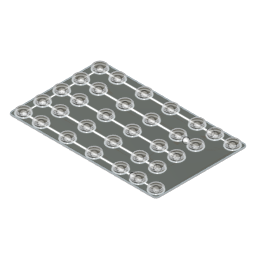
heliumv0.0.1prototype (Autodesk Fusion 360 design; units mm, degrees)
Autodesk Fusion 360 part; units mm, degrees
note: some values were not read from the file. Set by a fixed rule: which sketch regions a step uses.
sketch "Sketch1" plane through (0, 0, 0) normal (0, 0, 1) x (1, 0, 0)
  line L0 (2, 0) -> (98, 0)
  line L1 (100, 2) -> (100, 60)
  line L2 (98, 62) -> (2, 62)
  line L3 (0, 60) -> (0, 2)
  arc A0 (2, 62) -> (0, 60) centre (2, 60) ccw
  arc A1 (100, 60) -> (98, 62) centre (98, 60) ccw
  arc A2 (98, 0) -> (100, 2) centre (98, 2) ccw
  arc A3 (0, 2) -> (2, 0) centre (2, 2) ccw
  point P0 (100, 0)
  point P1 (0, 62)
  dimension "d1" = 100
  dimension "d2" = 62
  dimension "d3" = 2
  constraint horizontal L0
  constraint vertical L1
  constraint horizontal L2
  constraint vertical L3
  constraint coincident P1 L2
  constraint coincident P1 L3
  constraint tangent L2 A0
  constraint tangent L3 A0
  constraint tangent L1 A1
  constraint tangent L2 A1
  constraint equal A0 A1
  constraint coincident P0 L0
  constraint coincident P0 L1
  constraint tangent L0 A2
  constraint tangent L1 A2
  constraint equal A0 A2
  constraint coincident origin L0
  constraint coincident origin L3
  constraint tangent L0 A3
  constraint tangent L3 A3
  constraint equal A0 A3
  measures "d1" distance of origin P0
  measures "d2" distance of origin P1
  measures "d3" radius of A0
extrude "Extrude1" add sketch "Sketch1" along normal blind 0.5
sketch "Sketch2" plane through (0, 0, 0.5) normal (0, 0, 1) x (-1, 0, 0)
  arc A0 (0, -2) -> (-2, 0) centre (-2, -2) ccw
  line L0 (-2, 0) -> (-98, 0)
  arc A1 (-98, 0) -> (-100, -2) centre (-98, -2) ccw
  line L1 (-100, -2) -> (-100, -60)
  arc A2 (-100, -60) -> (-98, -62) centre (-98, -60) ccw
  line L2 (-98, -62) -> (-2, -62)
  arc A3 (-2, -62) -> (0, -60) centre (-2, -60) ccw
  line L3 (0, -60) -> (0, -2)
  line L4 (-5, -44) -> (-76.5418, -44)
  line L5 (-5, -44) -> (-17, -44)
  circle A4 centre (-5, -44) radius 4
  circle A5 centre (-17, -44) radius 4
  line L6 (-17, -44) -> (-35, -44)
  circle A6 centre (-35, -44) radius 4
  line L7 (-35, -44) -> (-40.411, -44)
  line L8 (-35, -44) -> (-53, -44)
  circle A7 centre (-53, -44) radius 4
  line L9 (-53, -44) -> (-59.411, -44)
  line L10 (-53, -44) -> (-71, -44)
  circle A8 centre (-71, -44) radius 4
  line L11 (-71, -44) -> (-83, -44)
  circle A9 centre (-83, -44) radius 4
  line L12 (-5, -44) -> (-5, -57)
  line L13 (-5, -57) -> (-79.7487, -57)
  circle A10 centre (-5, -57) radius 4
  line L14 (-5, -57) -> (-17, -57)
  line L15 (-17, -57) -> (-35, -57)
  line L16 (-35, -57) -> (-53, -57)
  line L17 (-53, -57) -> (-71, -57)
  line L18 (-71, -57) -> (-83, -57)
  circle A11 centre (-17, -57) radius 4
  circle A12 centre (-35, -57) radius 4
  circle A13 centre (-53, -57) radius 4
  circle A14 centre (-71, -57) radius 4
  circle A15 centre (-83, -57) radius 4
  line L19 (-5, -44) -> (-5, -31)
  line L20 (-5, -31) -> (-5, -18)
  circle A16 centre (-5, -31) radius 4
  circle A17 centre (-5, -18) radius 4
  line L21 (-5, -18) -> (-5, -5)
  circle A18 centre (-5, -5) radius 4
  line L22 (-5, -31) -> (-6.411, -31)
  line L23 (-6.411, -31) -> (-80.411, -31)
  line L24 (-5, -18) -> (-79.9028, -18)
  line L25 (-5, -5) -> (-79.411, -5)
  line L26 (-5, -31) -> (-17, -31)
  line L27 (-5, -18) -> (-17, -18)
  line L28 (-17, -31) -> (-17.411, -31)
  line L29 (-17, -31) -> (-35, -31)
  line L30 (-35, -31) -> (-53, -31)
  line L31 (-53, -31) -> (-71, -31)
  line L32 (-71, -31) -> (-83, -31)
  line L33 (-17, -18) -> (-35, -18)
  line L34 (-35, -18) -> (-53, -18)
  line L35 (-53, -18) -> (-71, -18)
  line L36 (-71, -18) -> (-83, -18)
  line L37 (-5, -5) -> (-17, -5)
  line L38 (-17, -5) -> (-35, -5)
  line L39 (-35, -5) -> (-53, -5)
  line L40 (-53, -5) -> (-71, -5)
  line L41 (-71, -5) -> (-83, -5)
  circle A19 centre (-17, -31) radius 4
  circle A20 centre (-35, -31) radius 4
  circle A21 centre (-53, -31) radius 4
  circle A22 centre (-71, -31) radius 4
  circle A23 centre (-83, -31) radius 4
  circle A24 centre (-83, -18) radius 4
  circle A25 centre (-71, -18) radius 4
  circle A26 centre (-53, -18) radius 4
  circle A27 centre (-35, -18) radius 4
  circle A28 centre (-17, -18) radius 4
  circle A29 centre (-17, -5) radius 4
  circle A30 centre (-35, -5) radius 4
  circle A31 centre (-53, -5) radius 4
  circle A32 centre (-71, -5) radius 4
  circle A33 centre (-83, -5) radius 4
  line L42 (-83, -5) -> (-95, -5)
  circle A34 centre (-95, -5) radius 4
  line L43 (-79.7487, -57) -> (-80, -57)
  line L44 (-83, -57) -> (-95, -57)
  circle A35 centre (-95, -57) radius 4
  dimension "d6" = 12
  dimension "d7" = 8
  dimension "d8" = 8
  dimension "d9" = 18
  dimension "d10" = 8
  dimension "d11" = 18
  dimension "d12" = 8
  dimension "d13" = 18
  dimension "d14" = 8
  dimension "d15" = 12
  dimension "d16" = 8
  dimension "d17" = 13
  dimension "d18" = 8
  dimension "d19" = 12
  dimension "d20" = 18
  dimension "d21" = 18
  dimension "d22" = 18
  dimension "d23" = 12
  dimension "d24" = 8
  dimension "d25" = 8
  dimension "d26" = 8
  dimension "d27" = 8
  dimension "d28" = 8
  dimension "d29" = 13
  dimension "d30" = 13
  dimension "d31" = 8
  dimension "d32" = 8
  dimension "d33" = 13
  dimension "d34" = 8
  dimension "d35" = 12
  dimension "d36" = 12
  dimension "d37" = 18
  dimension "d38" = 18
  dimension "d39" = 18
  dimension "d40" = 12
  dimension "d41" = 18
  dimension "d42" = 18
  dimension "d43" = 18
  dimension "d44" = 12
  dimension "d45" = 12
  dimension "d46" = 18
  dimension "d47" = 18
  dimension "d48" = 18
  dimension "d49" = 12
  dimension "d50" = 8
  dimension "d51" = 8
  dimension "d52" = 8
  dimension "d53" = 8
  dimension "d54" = 8
  dimension "d55" = 8
  dimension "d56" = 8
  dimension "d57" = 8
  dimension "d58" = 8
  dimension "d59" = 8
  dimension "d60" = 8
  dimension "d61" = 8
  dimension "d62" = 8
  dimension "d63" = 8
  dimension "d64" = 8
  dimension "d65" = 12
  dimension "d66" = 8
  dimension "d67" = 5
  dimension "d68" = 5
  dimension "d76" = 12
  dimension "d77" = 8
  constraint horizontal L4
  constraint perpendicular L3 L5
  constraint coincident L4.start L5.start
  constraint coincident L5.end A5.centre
  constraint parallel L4 L6
  constraint coincident L6.end A6.centre
  constraint coincident L4 L7.end
  constraint parallel L4 L7
  constraint parallel L4 L8
  constraint coincident L8.end A7.centre
  constraint coincident L4 L9.end
  constraint parallel L4 L10
  constraint coincident L10.end A8.centre
  constraint parallel L4 L11
  constraint coincident L11.end A9.centre
  constraint perpendicular L4 L12
  constraint perpendicular L12 L13
  constraint coincident L12.end L13.start
  constraint perpendicular L12 L14
  constraint parallel L13 L15
  constraint parallel L13 L16
  constraint parallel L13 L17
  constraint parallel L13 L18
  constraint coincident L14.end L15.start
  constraint coincident L15.end L16.start
  constraint coincident L16.end L17.start
  constraint coincident L17.end L18.start
  constraint coincident L18.end A15.centre
  constraint perpendicular L4 L19
  constraint parallel L19 L20
  constraint coincident L19.end L20.start
  constraint coincident L20.end A17.centre
  constraint parallel L20 L21
  constraint coincident L21.end A18.centre
  constraint perpendicular L19 L22
  constraint parallel L22 L23
  constraint perpendicular L21 L24
  constraint perpendicular L21 L25
  constraint perpendicular L19 L26
  constraint perpendicular L21 L27
  constraint coincident L23 L28.end
  constraint parallel L23 L29
  constraint parallel L23 L30
  constraint parallel L23 L31
  constraint parallel L23 L32
  constraint parallel L27 L33
  constraint parallel L24 L34
  constraint parallel L24 L35
  constraint parallel L24 L36
  constraint perpendicular L21 L37
  constraint parallel L25 L38
  constraint parallel L25 L39
  constraint parallel L25 L40
  constraint parallel L25 L41
  constraint coincident L26.end L28.start
  constraint coincident L29.end L30.start
  constraint coincident L30.end L31.start
  constraint coincident L31.end L32.start
  constraint coincident L32.end A23.centre
  constraint coincident L36.end A24.centre
  constraint coincident L35.end L36.start
  constraint coincident L34.end L35.start
  constraint coincident L33.end L34.start
  constraint coincident L27.end L33.start
  constraint coincident L37.end L38.start
  constraint coincident L38.end L39.start
  constraint coincident L39.end L40.start
  constraint coincident L40.end L41.start
  constraint coincident L41.end A33.centre
  constraint parallel L25 L42
  constraint coincident L42.end A34.centre
  constraint parallel L13 L43
  constraint parallel L13 L44
  constraint coincident L44.end A35.centre
  measures "d6" distance of L4.start L5.end
  measures "d7" diameter of A4
  measures "d8" diameter of A5
  measures "d9" distance of L5.end L6.end
  measures "d10" diameter of A6
  measures "d11" distance of L6.end L8.end
  measures "d12" diameter of A7
  measures "d13" distance of L8.end L10.end
  measures "d14" diameter of A8
  measures "d15" distance of L10.end L11.end
  measures "d16" diameter of A9
  measures "d17" distance of L4.start L12.end
  measures "d7" diameter of A10
  measures "d19" distance of L12.end L14.end
  measures "d20" distance of L14.end L15.end
  measures "d21" distance of L15.end L16.end
  measures "d22" distance of L16.end L17.end
  measures "d23" distance of L17.end L18.end
  measures "d24" diameter of A11
  measures "d25" diameter of A12
  measures "d26" diameter of A13
  measures "d27" diameter of A14
  measures "d28" diameter of A15
  measures "d29" distance of L4.start L19.end
  measures "d30" distance of L19.end L20.end
  measures "d31" diameter of A16
  measures "d32" diameter of A17
  measures "d33" distance of L20.end L21.end
  measures "d34" diameter of A18
  measures "d35" distance of L19.end L26.end
  measures "d36" distance of L20.end L27.end
  measures "d37" distance of L26.end L29.end
  measures "d38" distance of L29.end L30.end
  measures "d39" distance of L30.end L31.end
  measures "d40" distance of L31.end L32.end
  measures "d41" distance of L27.end L33.end
  measures "d42" distance of L33.end L34.end
  measures "d43" distance of L34.end L35.end
  measures "d44" distance of L35.end L36.end
  measures "d45" distance of L21.end L37.end
  measures "d46" distance of L37.end L38.end
  measures "d47" distance of L38.end L39.end
  measures "d48" distance of L39.end L40.end
  measures "d49" distance of L40.end L41.end
  measures "d50" diameter of A19
  measures "d51" diameter of A20
  measures "d52" diameter of A21
  measures "d53" diameter of A22
  measures "d54" diameter of A23
  measures "d55" diameter of A24
  measures "d56" diameter of A25
  measures "d57" diameter of A26
  measures "d58" diameter of A27
  measures "d59" diameter of A28
  measures "d60" diameter of A29
  measures "d61" diameter of A30
  measures "d62" diameter of A31
  measures "d63" diameter of A32
  measures "d64" diameter of A33
  measures "d65" distance of L41.end L42.end
  measures "d66" diameter of A34
  measures "d67" distance of L2 L12.end
  measures "d68" distance of L3 L12.end
  measures "d76" distance of L18.end L44.end
  measures "d77" diameter of A35
extrude "Extrude2" add sketch "Sketch2" along normal blind 2 contours L4 L5 A5 L6 | L4 L5 A5 L6 | L4 L6 A6 L7 L8 | L4 L6 A6 L7 L8 | L4 L8 A7 L9 L10 | L4 L8 A7 L9 L10 | L4 L10 A8 L11 | L4 L10 A8 L11 | L4 L5 A4 L12 | A4 L12 L19 | L4 L5 A4 L19 | A9 | L12 L13 A10 L14 | L12 L13 A10 L14 | L13 L14 L15 A11 | L13 L14 L15 A11 | L13 L15 L16 A12 | L13 L15 L16 A12 | L13 L16 L17 A13 | L13 L16 L17 A13 | L13 L17 L18 A14 | L13 L17 L18 A14 | L13 L18 A15 L43 L44 | L13 L18 A15 L43 L44 | L19 A16 L22 L23 L26 | L19 L20 A16 | L20 A16 L22 L23 L26 | L20 A17 L24 L27 | L20 A17 L21 | A17 L21 L24 L27 | L21 A18 L25 L37 | L21 A18 L25 L37 | L23 L26 L28 L29 A19 | L23 L26 L28 L29 A19 | L23 L29 L30 A20 | L23 L29 L30 A20 | L23 L30 L31 A21 | L23 L30 L31 A21 | L23 L31 L32 A22 | L23 L31 L32 A22 | L24 L27 L33 A28 | L24 L27 L33 A28 | L24 L33 L34 A27 | L24 L33 L34 A27 | L24 L34 L35 A26 | L24 L34 L35 A26 | L24 L35 L36 A25 | L24 L35 L36 A25 | L25 L37 L38 A29 | L25 L37 L38 A29 | L25 L38 L39 A30 | L25 L38 L39 A30 | L25 L39 L40 A31 | L25 L39 L40 A31 | L25 L40 L41 A32 | L25 L40 L41 A32 | L25 L41 A33 L42 | L25 L41 A33 L42 | A23 | A24 | A34 | A35
fillet "Fillet1" radius 0.5 32 edges at (8.7293, 58.4465, 2.5) (20.7293, 58.4465, 2.5) (38.7293, 58.4465, 2.5) (74.7293, 58.4465, 2.5) (56.7293, 58.4465, 2.5) (86.7293, 58.4465, 2.5) (86.7293, 45.4465, 2.5) (74.7293, 45.4465, 2.5) (56.7293, 45.4465, 2.5) (56.7293, 32.4465, 2.5) (74.7293, 32.4465, 2.5) (86.7293, 32.4465, 2.5) (86.7293, 19.4465, 2.5) (74.7293, 19.4465, 2.5) (86.7293, 6.4465, 2.5) (98.7293, 6.4465, 2.5) (74.7293, 6.4465, 2.5) (56.7293, 19.4465, 2.5) (56.7293, 6.4465, 2.5) (38.7293, 45.4465, 2.5) (38.7293, 32.4465, 2.5) (38.7293, 19.4465, 2.5) (38.7293, 6.4465, 2.5) (20.7293, 6.4465, 2.5) (20.7293, 19.4465, 2.5) (20.7293, 32.4465, 2.5) (20.7293, 45.4465, 2.5) (8.7293, 45.4465, 2.5) (8.7293, 32.4465, 2.5) (8.7293, 19.4465, 2.5) (8.7293, 6.4465, 2.5) (98.7293, 58.4465, 2.5)
